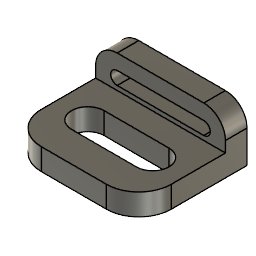
ex 2 (Autodesk Fusion 360 design; units mm, degrees)
part number: 2026-04-16-18-33-15-026
Autodesk Fusion 360 part; units mm, degrees
sketch "Sketch1" plane through (0, 0, 0) normal (0, 1, 0) x (1, 0, 0)
  line L0 (-30, -70) -> (50, -70)
  line L1 (70, -50) -> (70, -20)
  line L2 (70, -20) -> (-50, -20)
  line L3 (-50, -20) -> (-50, -50)
  arc A0 (50, -70) -> (70, -50) centre (50, -50) ccw
  arc A1 (-50, -50) -> (-30, -70) centre (-30, -50) ccw
  point P0 (-50, -70)
  point P1 (70, -70)
  dimension "d1" = 120
  dimension "d2" = 50
  dimension "d3" = 20
  dimension "d4" = 20
  constraint horizontal L0
  constraint vertical L1
  constraint horizontal L2
  constraint vertical L3
  constraint coincident P1 L0
  constraint coincident P1 L1
  constraint tangent L0 A0
  constraint tangent L1 A0
  constraint coincident P0 L0
  constraint coincident P0 L3
  constraint tangent L0 A1
  constraint tangent L3 A1
  measures "d1" distance of P0 P1
  measures "d2" distance of P0 L2.end
  measures "d3" radius of A0
  measures "d4" radius of A1
extrude "Extrude1" add sketch "Sketch1" along normal blind 20
sketch "Sketch2" plane through (0, 0, 0) normal (0, -1, 0) x (1, 0, 0)
  arc A0 (-30, 70) -> (-50, 50) centre (-30, 50) ccw
  line L0 (-50, 50) -> (-50, 20)
  line L1 (-50, 20) -> (70, 20)
  line L2 (70, 20) -> (70, 50)
  arc A1 (70, 50) -> (50, 70) centre (50, 50) ccw
  line L3 (50, 70) -> (-30, 70)
  line L4 (-30, 44) -> (50, 44)
  arc A2 (50, 44) -> (50, 56) centre (50, 50) ccw
  line L5 (50, 56) -> (-30, 56)
  arc A3 (-30, 56) -> (-30, 44) centre (-30, 50) ccw
  line L6 (-30, 50) -> (50, 50) construction
  dimension "d7" = 12
  constraint tangent L4 A2
  constraint tangent A2 L5
  constraint parallel L4 L5
  constraint tangent L5 A3
  constraint tangent L4 A3
  constraint horizontal L6
  measures "d7" diameter of A2
extrude "Extrude2" cut sketch "Sketch2" against normal blind 120 contours L4 A2 L5 A3
sketch "Sketch3" plane through (-50, 0, 0) normal (-1, 0, 0) x (0, -1, 0)
  line L0 (0, 20) -> (0, 50)
  line L1 (0, 50) -> (-20, 50)
  line L2 (-20, 50) -> (-20, 20)
  line L3 (-20, 20) -> (0, 20)
  line L4 (-20, 20) -> (80, 20)
  line L5 (80, 20) -> (80, 40)
  line L6 (80, 40) -> (-20, 40)
  line L7 (-20, 40) -> (-20, 20)
  dimension "d13" = 100
  dimension "d14" = 20
  constraint horizontal L4
  constraint vertical L5
  constraint horizontal L6
  constraint vertical L7
  constraint coincident L2.end L3.start
  measures "d13" distance of L2.end L4.end
  measures "d14" distance of L2.end L6.end
extrude "Extrude3" add sketch "Sketch3" against normal blind 120 contours L0 L4 L5 L6
fillet "Fillet1" radius 30 1 edges at (-50, -80, 30)
fillet "Fillet2" radius 30 1 edges at (70, -80, 30)
sketch "Sketch4" plane through (0, 0, 40) normal (0, 0, 1) x (-1, 0, 0)
  arc A0 (-40, 80) -> (-70, 50) centre (-40, 50) ccw
  line L0 (-70, 50) -> (-70, 0)
  line L1 (-70, 0) -> (50, 0)
  line L2 (50, 0) -> (50, 50)
  arc A1 (50, 50) -> (20, 80) centre (20, 50) ccw
  line L3 (20, 80) -> (-40, 80)
  line L4 (20, 52.1541) -> (-40, 52.1541)
  arc A2 (-40, 52.1541) -> (-40, 22.1541) centre (-40, 37.1541) ccw
  line L5 (-40, 22.1541) -> (20, 22.1541)
  arc A3 (20, 22.1541) -> (20, 52.1541) centre (20, 37.1541) ccw
  line L6 (20, 37.1541) -> (-40, 37.1541) construction
  dimension "d21" = 30
  dimension "d24" = 30
  constraint tangent L4 A2
  constraint tangent A2 L5
  constraint parallel L4 L5
  constraint tangent L5 A3
  constraint tangent L4 A3
  constraint perpendicular L2 L6
  measures "d21" diameter of A2
  measures "d24" distance of L0 A2.centre
extrude "Extrude4" cut sketch "Sketch4" against normal blind 80 contours L4 A2 L5 A3
